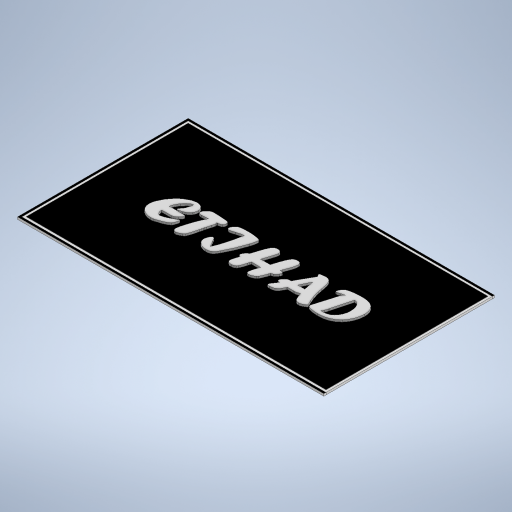
# Autodesk Inventor part: banner1
Saved by Autodesk Inventor 2024.1 (Build 281209000, 209)
## iProperties
Created: 2023-11-18
Part Number: banner1
Material: Generic
Document SubType Name: Modeling
Designer: ASUS
Density: 1 g/cm^3
Appearance: Default
Author: ASUS
Autodesk Inventor part; units mm, degrees
ref_plane "YZ Plane" through (0, 0, 0) normal (1, 0, 0) x (0, 1, 0)
ref_plane "XZ Plane" through (0, 0, 0) normal (0, 1, 0) x (-1, 0, 0)
ref_plane "XY Plane" through (0, 0, 0) normal (0, 0, 1) x (1, 0, 0)
sketch "Sketch1" plane through (0, 0, 0) normal (0, 1, 0) x (-1, 0, 0)
  line L0 (0, 0) -> (-71120, 0)
  line L1 (-71120, 0) -> (-71120, -19812)
  line L2 (-71120, -19812) -> (0, -19812)
  line L3 (0, -19812) -> (0, 0)
  line L4 (-254, -19558) -> (-70866, -19558)
  line L5 (-70866, -19558) -> (-70866, -254)
  line L6 (-70866, -254) -> (-254, -254)
  line L7 (-254, -254) -> (-254, -19558)
  line L8 (-35306, -19304) -> (-508, -19304)
  line L9 (-508, -19304) -> (-508, -508)
  line L10 (-508, -508) -> (-35306, -508)
  line L11 (-35306, -19304) -> (-35306, -508)
  line L12 (-6360.801, -11690.8525) -> (-20933.2375, -11690.8525) construction
  line L13 (-20933.2375, -11690.8525) -> (-20933.2375, -13635.6389) construction
  line L14 (-20933.2375, -13635.6389) -> (-6360.801, -13635.6389) construction
  line L15 (-6360.801, -13635.6389) -> (-6360.801, -11690.8525) construction
  line L16 (-41409.9422, -12220.6361) -> (-77079.4209, -12220.6361) construction
  line L17 (-77079.4209, -12220.6361) -> (-77079.4209, 7485.6525) construction
  line L18 (-77079.4209, 7485.6525) -> (-41409.9422, 7485.6525) construction
  line L19 (-41409.9422, 7485.6525) -> (-41409.9422, -12220.6361) construction
  line L20 (-9051.7121, -8799.8737) -> (-7938.0017, -8806.5427)
  line L21 (-7938.0017, -8806.5427) -> (-7938.0017, -8729.85)
  spline S0 degree 2 poles (-7938.0017, -8729.85) (-7938.0017, -8509.7755) (-8194.7553, -8146.3191) (-8351.475, -8146.3191) knots 0 0 0 1 2 2 2
  spline S1 degree 2 poles (-8351.475, -8146.3191) (-8508.1947, -8146.3191) (-9111.7324, -8379.7315) (-9495.1956, -8593.1371) knots 0 0 0 1 2 2 2
  line L22 (-9495.1956, -8593.1371) -> (-9601.8984, -8659.8263)
  spline S2 degree 2 poles (-9601.8984, -8659.8263) (-9711.9356, -8719.8466) (-9751.9492, -8749.8568) knots 0 0 0 1 1 1
  spline S3 degree 2 poles (-9751.9492, -8749.8568) (-9932.0102, -8863.2285) (-9978.6926, -8863.2285) knots 0 0 0 1 1 1
  spline S4 degree 2 poles (-9978.6926, -8863.2285) (-10032.044, -8863.2285) (-10032.044, -8763.1946) knots 0 0 0 1 1 1
  spline S5 degree 2 poles (-10032.044, -8763.1946) (-10032.044, -8653.1574) (-9952.0169, -8373.0625) (-9831.9763, -8112.9745) (-9768.6215, -8059.6231) knots 0 0 0 1 2 3 3 3
  spline S6 degree 2 poles (-9768.6215, -8059.6231) (-9595.2295, -7902.9034) (-8754.945, -7536.1125) (-8321.4648, -7432.7442) knots 0 0 0 1 2 2 2
  spline S7 degree 2 poles (-8321.4648, -7432.7442) (-8174.7485, -7402.734) (-8051.3734, -7402.734) knots 0 0 0 1 1 1
  spline S8 degree 2 poles (-8051.3734, -7402.734) (-7634.5656, -7402.734) (-6940.9974, -7739.5147) (-6560.8687, -8333.049) (-6560.8687, -8696.5054) knots 0 0 0 1 2 3 3 3
  spline S9 degree 2 poles (-6560.8687, -8696.5054) (-6560.8687, -8993.2725) (-6810.9534, -9713.5164) (-7261.1058, -10430.4258) (-7544.5351, -10720.524) knots 0 0 0 1 2 3 3 3
  spline S10 degree 2 poles (-7544.5351, -10720.524) (-7794.6198, -10977.2776) (-8404.8264, -11394.0854) (-8978.3539, -11620.8289) (-9221.7697, -11620.8289) knots 0 0 0 1 2 3 3 3
  spline S11 degree 2 poles (-9221.7697, -11620.8289) (-9598.5639, -11620.8289) (-10138.7468, -11190.6832) (-10138.7468, -10887.2471) knots 0 0 0 1 2 2 2
  spline S12 degree 2 poles (-10138.7468, -10887.2471) (-10138.7468, -10753.8687) (-10042.0474, -10437.0947) (-9958.6859, -10317.0541) knots 0 0 0 1 2 2 2
  spline S13 degree 2 poles (-9958.6859, -10317.0541) (-9871.9898, -10190.3445) (-9538.5436, -9946.9288) (-9328.4725, -9856.8983) knots 0 0 0 1 2 2 2
  spline S14 degree 2 poles (-9328.4725, -9856.8983) (-9075.0533, -9756.8644) (-8894.9924, -9756.8644) knots 0 0 0 1 1 1
  spline S15 degree 2 poles (-8894.9924, -9756.8644) (-8714.9314, -9756.8644) (-8714.9314, -9843.5604) knots 0 0 0 1 1 1
  spline S16 degree 2 poles (-8714.9314, -9843.5604) (-8714.9314, -9896.9118) (-8814.9653, -10006.9491) knots 0 0 0 1 1 1
  spline S17 degree 2 poles (-8814.9653, -10006.9491) (-8925.0025, -10103.6485) (-9025.0364, -10273.7061) knots 0 0 0 1 1 1
  spline S18 degree 2 poles (-9025.0364, -10273.7061) (-9121.7358, -10453.767) (-9268.4522, -10940.5985) (-9268.4522, -11077.3115) knots 0 0 0 1 2 2 2
  spline S19 degree 2 poles (-9268.4522, -11077.3115) (-9268.4522, -11190.6832) (-9201.7629, -11190.6832) knots 0 0 0 1 1 1
  spline S20 degree 2 poles (-9201.7629, -11190.6832) (-9095.0601, -11190.6832) (-8538.2049, -10720.524) (-8378.1507, -10493.7806) knots 0 0 0 1 2 2 2
  spline S21 degree 2 poles (-8378.1507, -10493.7806) (-8224.7654, -10280.375) (-8028.0322, -9836.8915) (-7994.6875, -9623.4859) knots 0 0 0 1 2 2 2
  line L23 (-7994.6875, -9623.4859) -> (-9625.2396, -9623.4859)
  spline S22 degree 2 poles (-9625.2396, -9623.4859) (-9895.3311, -9623.4859) (-9895.3311, -9486.773) knots 0 0 0 1 1 1
  spline S23 degree 2 poles (-9895.3311, -9486.773) (-9895.3311, -9356.7289) (-9595.2295, -9069.9652) knots 0 0 0 1 1 1
  spline S24 degree 2 poles (-9595.2295, -9069.9652) (-9298.4623, -8799.8737) (-9051.7121, -8799.8737) knots 0 0 0 1 1 1
  line L24 (-12172.7688, -9406.7459) -> (-12142.7587, -9273.3674)
  spline S25 degree 2 poles (-12142.7587, -9273.3674) (-12129.4208, -9206.6781) (-12102.7451, -9113.3132) (-12089.4073, -9043.2895) (-12079.4039, -9006.6104) knots 0 0 0 1 2 3 3 3
  spline S26 degree 2 poles (-12079.4039, -9006.6104) (-11859.3294, -8066.292) (-11725.9509, -7832.8796) knots 0 0 0 1 1 1
  spline S27 degree 2 poles (-11725.9509, -7832.8796) (-11665.9306, -7729.5113) (-11542.5555, -7646.1498) knots 0 0 0 1 1 1
  spline S28 degree 2 poles (-11542.5555, -7646.1498) (-11159.0923, -7396.0651) (-10939.0178, -7396.0651) knots 0 0 0 1 1 1
  spline S29 degree 2 poles (-10939.0178, -7396.0651) (-10785.6325, -7396.0651) (-10575.5614, -7619.4741) (-10575.5614, -7782.8627) knots 0 0 0 1 2 2 2
  spline S30 degree 2 poles (-10575.5614, -7782.8627) (-10575.5614, -8082.9643) (-10838.9839, -8886.5697) knots 0 0 0 1 1 1
  spline S31 degree 2 poles (-10838.9839, -8886.5697) (-10915.6765, -9143.3233) (-11049.055, -9520.1176) (-11232.4505, -9996.9457) (-11469.1973, -10533.7941) (-11515.8798, -10643.8314) knots 0 0 0 1 2 3 4 4 4
  spline S32 degree 2 poles (-11515.8798, -10643.8314) (-11115.7443, -10583.8111) (-10742.2845, -10583.8111) knots 0 0 0 1 1 1
  spline S33 degree 2 poles (-10742.2845, -10583.8111) (-10368.8247, -10583.8111) (-10368.8247, -10847.2336) knots 0 0 0 1 1 1
  spline S34 degree 2 poles (-10368.8247, -10847.2336) (-10368.8247, -11013.9567) (-10612.2405, -11270.7103) knots 0 0 0 1 1 1
  spline S35 degree 2 poles (-10612.2405, -11270.7103) (-10775.6291, -11440.7679) (-11055.724, -11570.8119) (-11255.7917, -11570.8119) knots 0 0 0 1 2 2 2
  spline S36 degree 2 poles (-11255.7917, -11570.8119) (-11382.5013, -11570.8119) (-11829.3192, -11554.1396) (-12222.7858, -11527.4639) knots 0 0 0 1 2 2 2
  line L25 (-12222.7858, -11527.4639) -> (-12309.4818, -11520.795)
  line L26 (-12309.4818, -11520.795) -> (-12389.5089, -11510.7916)
  spline S37 degree 2 poles (-12389.5089, -11510.7916) (-12726.2896, -11494.1193) (-12939.6952, -11444.1024) (-13016.3878, -11374.0787) knots 0 0 0 1 2 2 2
  spline S38 degree 2 poles (-13016.3878, -11374.0787) (-13076.4081, -11304.0549) (-13076.4081, -11214.0245) knots 0 0 0 1 1 1
  spline S39 degree 2 poles (-13076.4081, -11214.0245) (-13076.4081, -11117.3251) (-12999.7155, -10913.9228) (-12946.3641, -10863.9059) knots 0 0 0 1 2 2 2
  spline S40 degree 2 poles (-12946.3641, -10863.9059) (-12869.6715, -10780.5444) (-12519.5529, -10720.524) knots 0 0 0 1 1 1
  spline S41 degree 2 poles (-12519.5529, -10720.524) (-12489.5428, -10720.524) (-12456.1981, -10717.1896) knots 0 0 0 1 1 1
  line L27 (-12456.1981, -10717.1896) -> (-12392.8434, -10703.8517)
  spline S42 degree 2 poles (-12392.8434, -10703.8517) (-12466.2015, -10630.4935) (-12466.2015, -10540.4631) knots 0 0 0 1 1 1
  spline S43 degree 2 poles (-12466.2015, -10540.4631) (-12466.2015, -10457.1015) (-12382.84, -10173.6722) knots 0 0 0 1 1 1
  spline S44 degree 2 poles (-12382.84, -10173.6722) (-12352.8298, -10103.6485) (-12249.4615, -9713.5164) knots 0 0 0 1 1 1
  line L28 (-12249.4615, -9713.5164) -> (-12206.1135, -9530.121)
  line L29 (-12206.1135, -9530.121) -> (-12172.7688, -9406.7459)
  line L30 (-15307.1634, -11033.9635) -> (-15283.8222, -11033.9635)
  spline S45 degree 2 poles (-15283.8222, -11033.9635) (-15027.0686, -11033.9635) (-14430.1999, -10840.5647) knots 0 0 0 1 1 1
  spline S46 degree 2 poles (-14430.1999, -10840.5647) (-13990.0508, -10697.1828) (-13850.0034, -10697.1828) knots 0 0 0 1 1 1
  spline S47 degree 2 poles (-13850.0034, -10697.1828) (-13753.304, -10697.1828) (-13613.2566, -10820.5579) (-13613.2566, -10910.5884) knots 0 0 0 1 2 2 2
  spline S48 degree 2 poles (-13613.2566, -10910.5884) (-13613.2566, -11057.3047) (-13946.7028, -11487.4504) (-14113.4259, -11554.1396) knots 0 0 0 1 2 2 2
  spline S49 degree 2 poles (-14113.4259, -11554.1396) (-14360.1761, -11654.1735) (-15150.4437, -11654.1735) knots 0 0 0 1 1 1
  spline S50 degree 2 poles (-15150.4437, -11654.1735) (-15463.8832, -11654.1735) (-16097.431, -11594.1532) (-16534.2456, -11487.4504) (-16594.2659, -11427.43) knots 0 0 0 1 2 3 3 3
  spline S51 degree 2 poles (-16594.2659, -11427.43) (-16624.2761, -11397.4199) (-16624.2761, -11297.386) knots 0 0 0 1 1 1
  spline S52 degree 2 poles (-16624.2761, -11297.386) (-16624.2761, -11204.0211) (-16524.2422, -10723.8585) (-16454.2185, -10507.1184) knots 0 0 0 1 2 2 2
  spline S53 degree 2 poles (-16454.2185, -10507.1184) (-16024.0728, -9163.3301) (-15437.2075, -8089.6332) knots 0 0 0 1 1 1
  spline S54 degree 2 poles (-15437.2075, -8089.6332) (-15290.4911, -7819.5418) (-15020.3997, -7526.1091) (-14693.6224, -7402.734) (-14466.8789, -7402.734) knots 0 0 0 1 2 3 3 3
  spline S55 degree 2 poles (-14466.8789, -7402.734) (-14143.4361, -7402.734) (-13589.9153, -7649.4842) (-13269.807, -8072.9609) (-13269.807, -8326.3801) knots 0 0 0 1 2 3 3 3
  spline S56 degree 2 poles (-13269.807, -8326.3801) (-13269.807, -8503.1066) (-13419.8578, -8909.911) (-13513.2227, -9019.9482) knots 0 0 0 1 2 2 2
  spline S57 degree 2 poles (-13513.2227, -9019.9482) (-13559.9052, -9076.6341) (-13619.9255, -9076.6341) knots 0 0 0 1 1 1
  spline S58 degree 2 poles (-13619.9255, -9076.6341) (-13719.9594, -9076.6341) (-13896.6859, -8886.5697) (-14003.3887, -8659.8263) knots 0 0 0 1 2 2 2
  spline S59 degree 2 poles (-14003.3887, -8659.8263) (-14150.105, -8313.0422) (-14343.5038, -8082.9643) knots 0 0 0 1 1 1
  spline S60 degree 2 poles (-14343.5038, -8082.9643) (-14363.5106, -8056.2886) (-14436.8688, -7976.2615) knots 0 0 0 1 1 1
  spline S61 degree 2 poles (-14436.8688, -7976.2615) (-14580.2507, -8296.3699) (-14736.9704, -8706.5088) (-14837.0043, -9053.2929) knots 0 0 0 1 2 2 2
  spline S62 degree 2 poles (-14837.0043, -9053.2929) (-14907.028, -9270.0329) (-15073.7511, -9900.2463) knots 0 0 0 1 1 1
  spline S63 degree 2 poles (-15073.7511, -9900.2463) (-15207.1296, -10427.0913) (-15307.1634, -11033.9635) knots 0 0 0 1 1 1
  line L31 (-18364.8654, -8793.2048) -> (-18301.5106, -8589.8026)
  spline S64 degree 2 poles (-18301.5106, -8589.8026) (-18288.1728, -8523.1134) (-18254.8282, -8409.7416) knots 0 0 0 1 1 1
  spline S65 degree 2 poles (-18254.8282, -8409.7416) (-18088.105, -7836.2141) (-17981.4022, -7656.1531) knots 0 0 0 1 1 1
  spline S66 degree 2 poles (-17981.4022, -7656.1531) (-17958.061, -7619.4741) (-17901.3751, -7549.4503) knots 0 0 0 1 1 1
  spline S67 degree 2 poles (-17901.3751, -7549.4503) (-17704.6419, -7369.3894) (-17421.2126, -7369.3894) knots 0 0 0 1 1 1
  spline S68 degree 2 poles (-17421.2126, -7369.3894) (-17194.4691, -7369.3894) (-16921.0432, -7566.1227) (-16921.0432, -7722.8424) knots 0 0 0 1 2 2 2
  spline S69 degree 2 poles (-16921.0432, -7722.8424) (-16921.0432, -7836.2141) (-17081.0974, -8416.4106) (-17177.7968, -8679.8331) knots 0 0 0 1 2 2 2
  spline S70 degree 2 poles (-17177.7968, -8679.8331) (-16937.7155, -8726.5156) (-16937.7155, -8883.2353) knots 0 0 0 1 1 1
  spline S71 degree 2 poles (-16937.7155, -8883.2353) (-16937.7155, -8996.607) (-17087.7663, -9280.0363) (-17314.5098, -9506.7797) (-17421.2126, -9540.1244) knots 0 0 0 1 2 3 3 3
  spline S72 degree 2 poles (-17421.2126, -9540.1244) (-17467.895, -9670.1684) (-17597.9391, -10090.3107) knots 0 0 0 1 1 1
  spline S73 degree 2 poles (-17597.9391, -10090.3107) (-17884.7028, -11003.9533) (-18064.7638, -11314.0583) knots 0 0 0 1 1 1
  spline S74 degree 2 poles (-18064.7638, -11314.0583) (-18138.122, -11417.4267) (-18191.4734, -11474.1125) knots 0 0 0 1 1 1
  spline S75 degree 2 poles (-18191.4734, -11474.1125) (-18348.1931, -11624.1633) (-18594.9433, -11624.1633) knots 0 0 0 1 1 1
  spline S76 degree 2 poles (-18594.9433, -11624.1633) (-18748.3286, -11624.1633) (-18981.7409, -11517.4605) (-19105.116, -11330.7306) (-19105.116, -11207.3555) knots 0 0 0 1 2 3 3 3
  spline S77 degree 2 poles (-19105.116, -11207.3555) (-19105.116, -11033.9635) (-18671.6359, -9746.861) knots 0 0 0 1 1 1
  spline S78 degree 2 poles (-18671.6359, -9746.861) (-18664.967, -9726.8543) (-18638.2913, -9643.4927) (-18624.9535, -9610.1481) knots 0 0 0 1 2 2 2
  line L32 (-18624.9535, -9610.1481) -> (-18614.9501, -9586.8068)
  line L33 (-18614.9501, -9586.8068) -> (-19735.3294, -9610.1481)
  line L34 (-19735.3294, -9610.1481) -> (-19788.6808, -9803.5469)
  spline S79 degree 2 poles (-19788.6808, -9803.5469) (-19885.3802, -10113.6519) (-20092.1169, -10720.524) (-20242.1677, -11087.3149) (-20395.553, -11367.4097) (-20462.2422, -11437.4334) knots 0 0 0 1 2 3 4 4 4
  spline S80 degree 2 poles (-20462.2422, -11437.4334) (-20622.2964, -11610.8255) (-20902.3912, -11610.8255) knots 0 0 0 1 1 1
  spline S81 degree 2 poles (-20902.3912, -11610.8255) (-21375.8849, -11610.8255) (-21375.8849, -11200.6866) knots 0 0 0 1 1 1
  spline S82 degree 2 poles (-21375.8849, -11200.6866) (-21375.8849, -10813.889) (-20962.4116, -9790.209) knots 0 0 0 1 1 1
  spline S83 degree 2 poles (-20962.4116, -9790.209) (-20902.3912, -9636.8238) (-20892.3879, -9603.4791) knots 0 0 0 1 1 1
  spline S84 degree 2 poles (-20892.3879, -9603.4791) (-20902.3912, -9606.8136) (-20922.398, -9610.1481) (-20932.4014, -9610.1481) knots 0 0 0 1 2 2 2
  spline S85 degree 2 poles (-20932.4014, -9610.1481) (-21099.1245, -9610.1481) (-21289.1889, -9490.1074) (-21289.1889, -9390.0736) knots 0 0 0 1 2 2 2
  spline S86 degree 2 poles (-21289.1889, -9390.0736) (-21289.1889, -9323.3843) (-21205.8273, -9196.6747) knots 0 0 0 1 1 1
  spline S87 degree 2 poles (-21205.8273, -9196.6747) (-21125.8002, -9073.2996) (-20939.0703, -8879.9008) (-20872.3811, -8839.8873) knots 0 0 0 1 2 2 2
  spline S88 degree 2 poles (-20872.3811, -8839.8873) (-20809.0263, -8806.5427) (-20625.6309, -8769.8636) knots 0 0 0 1 1 1
  line L35 (-20625.6309, -8769.8636) -> (-20612.293, -8719.8466)
  spline S89 degree 2 poles (-20612.293, -8719.8466) (-20592.2862, -8676.4986) (-20548.9382, -8553.1235) knots 0 0 0 1 1 1
  spline S90 degree 2 poles (-20548.9382, -8553.1235) (-20485.5835, -8376.397) (-20352.205, -8019.6095) (-20262.1745, -7822.8763) (-20218.8265, -7756.187) knots 0 0 0 1 2 3 3 3
  spline S91 degree 2 poles (-20218.8265, -7756.187) (-20168.8095, -7682.8288) (-20102.1203, -7632.8119) knots 0 0 0 1 1 1
  spline S92 degree 2 poles (-20102.1203, -7632.8119) (-19955.4039, -7519.4402) (-19575.2752, -7376.0583) (-19451.9001, -7376.0583) knots 0 0 0 1 2 2 2
  spline S93 degree 2 poles (-19451.9001, -7376.0583) (-19305.1838, -7376.0583) (-19141.7951, -7516.1057) (-19141.7951, -7642.8153) knots 0 0 0 1 2 2 2
  spline S94 degree 2 poles (-19141.7951, -7642.8153) (-19141.7951, -7862.8898) (-19371.873, -8553.1235) knots 0 0 0 1 1 1
  spline S95 degree 2 poles (-19371.873, -8553.1235) (-19425.2244, -8706.5088) (-19445.2312, -8776.5325) knots 0 0 0 1 1 1
  line L36 (-19445.2312, -8776.5325) -> (-18364.8654, -8793.2048)
  line L37 (-23676.6639, -11133.9974) -> (-23489.934, -11467.4436)
  spline S96 degree 2 poles (-23489.934, -11467.4436) (-23559.9577, -11524.1295) (-23619.9781, -11544.1362) knots 0 0 0 1 1 1
  spline S97 degree 2 poles (-23619.9781, -11544.1362) (-23856.7249, -11624.1633) (-24186.8366, -11624.1633) knots 0 0 0 1 1 1
  spline S98 degree 2 poles (-24186.8366, -11624.1633) (-24523.6173, -11624.1633) (-24707.0128, -11430.7645) knots 0 0 0 1 1 1
  spline S99 degree 2 poles (-24707.0128, -11430.7645) (-24863.7325, -11264.0414) (-25063.8002, -10660.5037) (-25150.4963, -10103.6485) knots 0 0 0 1 2 2 2
  spline S100 degree 2 poles (-25150.4963, -10103.6485) (-25197.1787, -9820.2192) (-25230.5234, -9676.8373) knots 0 0 0 1 1 1
  spline S101 degree 2 poles (-25230.5234, -9676.8373) (-25337.2262, -9276.7018) (-25407.2499, -9056.6273) (-25500.6148, -8813.2116) knots 0 0 0 1 2 2 2
  spline S102 degree 2 poles (-25500.6148, -8813.2116) (-25530.625, -8743.1879) (-25630.6588, -8489.7687) (-25677.3413, -8379.7315) knots 0 0 0 1 2 2 2
  spline S103 degree 2 poles (-25677.3413, -8379.7315) (-25777.3752, -8142.9846) (-25980.7774, -7752.8526) knots 0 0 0 1 1 1
  spline S104 degree 2 poles (-25980.7774, -7752.8526) (-25724.0238, -7572.7916) (-25370.5708, -7412.7374) (-25223.8544, -7412.7374) knots 0 0 0 1 2 2 2
  spline S105 degree 2 poles (-25223.8544, -7412.7374) (-25043.7935, -7412.7374) (-24803.7122, -7552.7848) (-24707.0128, -7706.1701) knots 0 0 0 1 2 2 2
  spline S106 degree 2 poles (-24707.0128, -7706.1701) (-24590.3066, -7912.9067) (-24473.6004, -8269.6942) knots 0 0 0 1 1 1
  spline S107 degree 2 poles (-24473.6004, -8269.6942) (-24463.597, -8303.0388) (-24430.2524, -8406.4072) (-24406.9112, -8469.762) knots 0 0 0 1 2 2 2
  spline S108 degree 2 poles (-24406.9112, -8469.762) (-24050.1237, -8319.7111) (-23853.3904, -8319.7111) knots 0 0 0 1 1 1
  spline S109 degree 2 poles (-23853.3904, -8319.7111) (-23740.0187, -8319.7111) (-23656.6571, -8326.3801) knots 0 0 0 1 1 1
  spline S110 degree 2 poles (-23656.6571, -8326.3801) (-23586.6334, -8329.7145) (-23003.1025, -8343.0524) knots 0 0 0 1 1 1
  line L38 (-23003.1025, -8343.0524) -> (-22976.4268, -8283.0321)
  spline S111 degree 2 poles (-22976.4268, -8283.0321) (-22806.3692, -7926.2446) (-22516.271, -7552.7848) (-22132.8078, -7399.3995) (-21846.0441, -7399.3995) knots 0 0 0 1 2 3 3 3
  spline S112 degree 2 poles (-21846.0441, -7399.3995) (-21682.6554, -7399.3995) (-21542.608, -7472.7577) (-21542.608, -7556.1193) knots 0 0 0 1 2 2 2
  spline S113 degree 2 poles (-21542.608, -7556.1193) (-21542.608, -7656.1531) (-21879.3887, -8109.64) knots 0 0 0 1 1 1
  spline S114 degree 2 poles (-21879.3887, -8109.64) (-21996.0949, -8269.6942) (-22056.1152, -8359.7247) knots 0 0 0 1 1 1
  spline S115 degree 2 poles (-22056.1152, -8359.7247) (-21736.0068, -8419.745) (-21736.0068, -8586.4681) knots 0 0 0 1 1 1
  spline S116 degree 2 poles (-21736.0068, -8586.4681) (-21736.0068, -8719.8466) (-21992.7604, -8986.6036) knots 0 0 0 1 1 1
  spline S117 degree 2 poles (-21992.7604, -8986.6036) (-22112.8011, -9113.3132) (-22322.8722, -9183.3369) (-22586.2947, -9186.6714) knots 0 0 0 1 2 2 2
  spline S118 degree 2 poles (-22586.2947, -9186.6714) (-22829.7105, -9633.4893) (-22963.089, -9880.2395) (-23176.4946, -10257.0338) (-23446.586, -10733.8619) (-23676.6639, -11133.9974) knots 0 0 0 1 2 3 4 4 4
  line L39 (-23940.0864, -10327.0575) -> (-23383.2312, -9146.6578)
  line L40 (-23383.2312, -9146.6578) -> (-24206.8434, -9146.6578)
  line L41 (-24206.8434, -9146.6578) -> (-23950.0898, -10327.0575)
  line L42 (-23950.0898, -10327.0575) -> (-23940.0864, -10327.0575)
  line L43 (-26137.4971, -7919.5757) -> (-26864.4099, -10367.071)
  spline S119 degree 2 poles (-26864.4099, -10367.071) (-26941.1025, -10650.5003) (-27024.4641, -10767.2065) knots 0 0 0 1 1 1
  spline S120 degree 2 poles (-27024.4641, -10767.2065) (-27077.8155, -10833.8958) (-27161.1771, -10880.5782) knots 0 0 0 1 1 1
  line L44 (-27161.1771, -10880.5782) -> (-27161.1771, -10890.5816)
  line L45 (-27161.1771, -10890.5816) -> (-27117.829, -10890.5816)
  spline S121 degree 2 poles (-27117.829, -10890.5816) (-27031.133, -10890.5816) (-26751.0382, -10790.5477) knots 0 0 0 1 1 1
  spline S122 degree 2 poles (-26751.0382, -10790.5477) (-26444.2677, -10683.8449) (-26327.5615, -10683.8449) knots 0 0 0 1 1 1
  spline S123 degree 2 poles (-26327.5615, -10683.8449) (-26267.5411, -10683.8449) (-26220.8587, -10727.193) (-26220.8587, -10777.2099) knots 0 0 0 1 2 2 2
  spline S124 degree 2 poles (-26220.8587, -10777.2099) (-26220.8587, -10900.585) (-26357.5716, -11190.6832) (-26577.6461, -11420.7611) (-26694.3523, -11470.7781) knots 0 0 0 1 2 3 3 3
  spline S125 degree 2 poles (-26694.3523, -11470.7781) (-26957.7749, -11574.1464) (-27864.7486, -11690.8526) (-28398.2626, -11690.8526) knots 0 0 0 1 2 2 2
  spline S126 degree 2 poles (-28398.2626, -11690.8526) (-28971.7901, -11690.8526) (-29775.3955, -11330.7306) (-30192.2033, -10623.8246) (-30192.2033, -10123.6553) knots 0 0 0 1 2 3 3 3
  spline S127 degree 2 poles (-30192.2033, -10123.6553) (-30192.2033, -9620.1515) (-29792.0678, -8599.806) (-29465.2905, -8253.0219) knots 0 0 0 1 2 2 2
  spline S128 degree 2 poles (-29465.2905, -8253.0219) (-28695.0297, -7436.0786) (-27404.5928, -7436.0786) knots 0 0 0 1 1 1
  spline S129 degree 2 poles (-27404.5928, -7436.0786) (-26991.1195, -7436.0786) (-26304.2202, -7569.4571) (-26194.183, -7669.491) knots 0 0 0 1 2 2 2
  spline S130 degree 2 poles (-26194.183, -7669.491) (-26124.1593, -7722.8424) (-26124.1593, -7829.5452) knots 0 0 0 1 1 1
  spline S131 degree 2 poles (-26124.1593, -7829.5452) (-26124.1593, -7856.2209) (-26137.4971, -7919.5757) knots 0 0 0 1 1 1
  line L46 (-28201.5293, -10953.9364) -> (-27584.6538, -8636.4851)
  spline S132 degree 2 poles (-27584.6538, -8636.4851) (-27577.9848, -8613.1438) (-27561.3125, -8523.1134) knots 0 0 0 1 1 1
  spline S133 degree 2 poles (-27561.3125, -8523.1134) (-27504.6267, -8283.0321) (-27434.603, -8149.6536) knots 0 0 0 1 1 1
  spline S134 degree 2 poles (-27434.603, -8149.6536) (-27387.9205, -8049.6197) (-27281.2177, -7919.5757) knots 0 0 0 1 1 1
  spline S135 degree 2 poles (-27281.2177, -7919.5757) (-27367.9137, -7912.9067) (-27477.951, -7912.9067) knots 0 0 0 1 1 1
  spline S136 degree 2 poles (-27477.951, -7912.9067) (-27744.708, -7912.9067) (-28098.161, -7982.9305) (-28401.597, -8152.988) (-28534.9755, -8289.701) knots 0 0 0 1 2 3 3 3
  spline S137 degree 2 poles (-28534.9755, -8289.701) (-28788.3947, -8546.4546) (-29058.4861, -9230.0194) (-29058.4861, -9630.1548) knots 0 0 0 1 2 2 2
  spline S138 degree 2 poles (-29058.4861, -9630.1548) (-29058.4861, -9996.9457) (-28841.7461, -10593.8145) (-28451.614, -10937.2641) (-28201.5293, -10953.9364) knots 0 0 0 1 2 3 3 3
  spline S139 degree 2 poles (-42991.5474, -7910.8463) (-42539.6602, -7910.8463) (-41905.6692, -8099.6946) (-41625.769, -8234.5863) knots 0 0 0 1 2 2 2
  line L47 (-41625.769, -8234.5863) -> (-41625.769, -8929.2786)
  line L48 (-41625.769, -8929.2786) -> (-41666.2365, -8929.2786)
  spline S140 degree 2 poles (-41666.2365, -8929.2786) (-41939.3922, -8672.9844) (-42630.7121, -8389.7118) (-42951.0799, -8389.7118) knots 0 0 0 1 2 2 2
  spline S141 degree 2 poles (-42951.0799, -8389.7118) (-43409.7117, -8389.7118) (-43878.4604, -8770.7809) (-43878.4604, -9084.4041) knots 0 0 0 1 2 2 2
  spline S142 degree 2 poles (-43878.4604, -9084.4041) (-43878.4604, -9333.9537) (-43632.283, -9644.2046) (-43365.8719, -9721.7673) knots 0 0 0 1 2 2 2
  spline S143 degree 2 poles (-43365.8719, -9721.7673) (-43173.6512, -9775.724) (-42853.2834, -9849.9145) (-42613.8507, -9910.6157) knots 0 0 0 1 2 2 2
  spline S144 degree 2 poles (-42613.8507, -9910.6157) (-42398.024, -9967.9447) (-42057.4224, -10139.9316) (-41925.903, -10278.1956) knots 0 0 0 1 2 2 2
  spline S145 degree 2 poles (-41925.903, -10278.1956) (-41797.7559, -10416.4596) (-41656.1196, -10787.4118) (-41656.1196, -11030.2169) knots 0 0 0 1 2 2 2
  spline S146 degree 2 poles (-41656.1196, -11030.2169) (-41656.1196, -11536.0607) (-42445.236, -12220.6361) (-43055.621, -12220.6361) knots 0 0 0 1 2 2 2
  spline S147 degree 2 poles (-43055.621, -12220.6361) (-43406.3394, -12220.6361) (-44026.8413, -12082.3721) (-44293.2524, -11950.8527) knots 0 0 0 1 2 2 2
  line L49 (-44293.2524, -11950.8527) -> (-44293.2524, -11289.8834)
  line L50 (-44293.2524, -11289.8834) -> (-44252.7849, -11289.8834)
  spline S148 degree 2 poles (-44252.7849, -11289.8834) (-44053.8196, -11471.9872) (-43433.3178, -11741.7706) (-43092.7162, -11741.7706) knots 0 0 0 1 2 2 2
  spline S149 degree 2 poles (-43092.7162, -11741.7706) (-42708.2749, -11741.7706) (-42232.7816, -11380.9353) (-42232.7816, -11087.5458) knots 0 0 0 1 2 2 2
  spline S150 degree 2 poles (-42232.7816, -11087.5458) (-42232.7816, -10824.507) (-42512.6819, -10510.8838) (-42775.7207, -10440.0657) knots 0 0 0 1 2 2 2
  spline S151 degree 2 poles (-42775.7207, -10440.0657) (-42951.0799, -10392.8536) (-43460.2961, -10271.451) (-43628.9107, -10220.8666) knots 0 0 0 1 2 2 2
  spline S152 degree 2 poles (-43628.9107, -10220.8666) (-44057.1919, -10089.3472) (-44455.1224, -9559.8973) (-44455.1224, -9172.0837) knots 0 0 0 1 2 2 2
  spline S153 degree 2 poles (-44455.1224, -9172.0837) (-44455.1224, -8925.9063) (-44256.1571, -8453.7854) (-44077.4256, -8288.543) knots 0 0 0 1 2 2 2
  spline S154 degree 2 poles (-44077.4256, -8288.543) (-43878.4604, -8106.4392) (-43372.6165, -7910.8463) (-42991.5474, -7910.8463) knots 0 0 0 1 2 2 2
  line L51 (-45989.5155, -7985.0367) -> (-45989.5155, -11654.091)
  line L52 (-45989.5155, -11654.091) -> (-44593.3864, -11654.091)
  line L53 (-44593.3864, -11654.091) -> (-44593.3864, -12146.4457)
  line L54 (-44593.3864, -12146.4457) -> (-47938.7006, -12146.4457)
  line L55 (-47938.7006, -12146.4457) -> (-47938.7006, -11654.091)
  line L56 (-47938.7006, -11654.091) -> (-46542.5715, -11654.091)
  line L57 (-46542.5715, -11654.091) -> (-46542.5715, -7985.0367)
  line L58 (-46542.5715, -7985.0367) -> (-45989.5155, -7985.0367)
  line L59 (-47911.7223, -7985.0367) -> (-49314.596, -12146.4457)
  line L60 (-49314.596, -12146.4457) -> (-49995.799, -12146.4457)
  line L61 (-49995.799, -12146.4457) -> (-51398.6727, -7985.0367)
  line L62 (-51398.6727, -7985.0367) -> (-50815.2661, -7985.0367)
  line L63 (-50815.2661, -7985.0367) -> (-50437.5694, -9148.4776)
  line L64 (-50437.5694, -9148.4776) -> (-48849.2196, -9148.4776)
  line L65 (-48849.2196, -9148.4776) -> (-48471.5228, -7985.0367)
  line L66 (-48471.5228, -7985.0367) -> (-47911.7223, -7985.0367)
  line L67 (-50285.8162, -9620.5986) -> (-49641.7083, -11579.9005)
  line L68 (-49641.7083, -11579.9005) -> (-49000.9727, -9620.5986)
  line L69 (-49000.9727, -9620.5986) -> (-50285.8162, -9620.5986)
  spline S155 degree 2 poles (-55074.4716, -10062.3689) (-55074.4716, -9492.4515) (-54612.4675, -8575.1879) (-54224.6539, -8318.8936) knots 0 0 0 1 2 2 2
  spline S156 degree 2 poles (-54224.6539, -8318.8936) (-53907.6584, -8119.9284) (-53256.8059, -7985.0367) (-52750.9621, -7985.0367) knots 0 0 0 1 2 2 2
  line L70 (-52750.9621, -7985.0367) -> (-51793.231, -7985.0367)
  line L71 (-51793.231, -7985.0367) -> (-51793.231, -12146.4457)
  line L72 (-51793.231, -12146.4457) -> (-52740.8452, -12146.4457)
  spline S157 degree 2 poles (-52740.8452, -12146.4457) (-53327.6241, -12146.4457) (-53995.338, -11971.0865) (-54231.3985, -11815.961) knots 0 0 0 1 2 2 2
  spline S158 degree 2 poles (-54231.3985, -11815.961) (-54632.7013, -11549.5499) (-55074.4716, -10669.3816) (-55074.4716, -10062.3689) knots 0 0 0 1 2 2 2
  spline S159 degree 2 poles (-54497.8096, -10069.1135) (-54497.8096, -10547.979) (-54180.8141, -11225.8098) (-53867.1909, -11418.0305) knots 0 0 0 1 2 2 2
  spline S160 degree 2 poles (-53867.1909, -11418.0305) (-53644.6196, -11549.5499) (-53142.148, -11667.5801) (-52767.8235, -11667.5801) knots 0 0 0 1 2 2 2
  line L73 (-52767.8235, -11667.5801) -> (-52346.287, -11667.5801)
  line L74 (-52346.287, -11667.5801) -> (-52346.287, -8463.9022)
  line L75 (-52346.287, -8463.9022) -> (-52767.8235, -8463.9022)
  spline S161 degree 2 poles (-52767.8235, -8463.9022) (-53135.4034, -8463.9022) (-53691.8317, -8581.9325) (-53917.7753, -8740.4302) knots 0 0 0 1 2 2 2
  spline S162 degree 2 poles (-53917.7753, -8740.4302) (-54207.7924, -8936.0232) (-54497.8096, -9583.5034) (-54497.8096, -10069.1135) knots 0 0 0 1 2 2 2
  line L76 (-57124.8255, -7985.0367) -> (-55512.8696, -7985.0367)
  line L77 (-55512.8696, -7985.0367) -> (-55512.8696, -8409.9455)
  line L78 (-55512.8696, -8409.9455) -> (-56042.3196, -8409.9455)
  line L79 (-56042.3196, -8409.9455) -> (-56042.3196, -11721.5368)
  line L80 (-56042.3196, -11721.5368) -> (-55512.8696, -11721.5368)
  line L81 (-55512.8696, -11721.5368) -> (-55512.8696, -12146.4457)
  line L82 (-55512.8696, -12146.4457) -> (-57124.8255, -12146.4457)
  line L83 (-57124.8255, -12146.4457) -> (-57124.8255, -11721.5368)
  line L84 (-57124.8255, -11721.5368) -> (-56595.3756, -11721.5368)
  line L85 (-56595.3756, -11721.5368) -> (-56595.3756, -8409.9455)
  line L86 (-56595.3756, -8409.9455) -> (-57124.8255, -8409.9455)
  line L87 (-57124.8255, -8409.9455) -> (-57124.8255, -7985.0367)
  spline S163 degree 2 poles (-59262.859, -7897.3571) (-58895.2791, -7897.3571) (-58348.9677, -8089.5778) (-58156.747, -8281.7984) knots 0 0 0 1 2 2 2
  spline S164 degree 2 poles (-58156.747, -8281.7984) (-57937.548, -8497.6252) (-57758.8165, -9104.6378) (-57758.8165, -9549.7804) knots 0 0 0 1 2 2 2
  line L88 (-57758.8165, -9549.7804) -> (-57758.8165, -12146.4457)
  line L89 (-57758.8165, -12146.4457) -> (-58311.8725, -12146.4457)
  line L90 (-58311.8725, -12146.4457) -> (-58311.8725, -9549.7804)
  spline S165 degree 2 poles (-58311.8725, -9549.7804) (-58311.8725, -9259.7633) (-58386.0629, -8868.5773) (-58490.604, -8710.0796) knots 0 0 0 1 2 2 2
  spline S166 degree 2 poles (-58490.604, -8710.0796) (-58601.8896, -8541.465) (-58986.331, -8369.478) (-59262.859, -8369.478) knots 0 0 0 1 2 2 2
  spline S167 degree 2 poles (-59262.859, -8369.478) (-59522.5255, -8369.478) (-59927.2006, -8541.465) (-60038.4862, -8710.0796) knots 0 0 0 1 2 2 2
  spline S168 degree 2 poles (-60038.4862, -8710.0796) (-60143.0273, -8868.5773) (-60217.2177, -9256.391) (-60217.2177, -9536.2913) knots 0 0 0 1 2 2 2
  line L91 (-60217.2177, -9536.2913) -> (-60217.2177, -12146.4457)
  line L92 (-60217.2177, -12146.4457) -> (-60770.2737, -12146.4457)
  line L93 (-60770.2737, -12146.4457) -> (-60770.2737, -9549.7804)
  spline S169 degree 2 poles (-60770.2737, -9549.7804) (-60770.2737, -9114.7547) (-60594.9145, -8494.2529) (-60372.3432, -8281.7984) knots 0 0 0 1 2 2 2
  spline S170 degree 2 poles (-60372.3432, -8281.7984) (-60173.3779, -8086.2055) (-59647.3003, -7897.3571) (-59262.859, -7897.3571) knots 0 0 0 1 2 2 2
  line L94 (-65130.648, -7985.0367) -> (-64577.592, -7985.0367)
  line L95 (-64577.592, -7985.0367) -> (-64577.592, -11569.7837)
  line L96 (-64577.592, -11569.7837) -> (-63491.7138, -9131.6162)
  line L97 (-63491.7138, -9131.6162) -> (-63154.4845, -9131.6162)
  line L98 (-63154.4845, -9131.6162) -> (-62078.7232, -11569.7837)
  line L99 (-62078.7232, -11569.7837) -> (-62078.7232, -7985.0367)
  line L100 (-62078.7232, -7985.0367) -> (-61562.7625, -7985.0367)
  line L101 (-61562.7625, -7985.0367) -> (-61562.7625, -12146.4457)
  line L102 (-61562.7625, -12146.4457) -> (-62318.156, -12146.4457)
  line L103 (-62318.156, -12146.4457) -> (-63356.8221, -9829.6807)
  line L104 (-63356.8221, -9829.6807) -> (-64361.7653, -12146.4457)
  line L105 (-64361.7653, -12146.4457) -> (-65130.648, -12146.4457)
  line L106 (-65130.648, -12146.4457) -> (-65130.648, -7985.0367)
  dimension "d3" = 19812
  constraints: 24 end point, 5 parallel, 2 perpendicular, 1 horizontal, 7 other
  measures "d3" distance of L0.end L1.end
extrude "Extrusion1" add sketch "Sketch1" along normal blind 508 contours L20 L21 S0 S1 L22 S2 S3 S4 S5 S6 S7 S8 S9 S10 S11 S12 S13 S14 S15 S16 S17 S18 S19 S20 S21 L23 S22 S23 S24 | L24 S25 S26 S27 S28 S29 S30 S31 S32 S33 S34 S35 S36 L25 L26 S37 S38 S39 S40 S41 L27 S42 S43 S44 L28 L29 | L30 S45 S46 S47 S48 S49 S50 S51 S52 S53 S54 S55 S56 S57 S58 S59 S60 S61 S62 S63 | L31 S64 S65 S66 S67 S68 S69 S70 S71 S72 S73 S74 S75 S76 S77 S78 L32 L33 L34 S79 S80 S81 S82 S83 S84 S85 S86 S87 S88 L35 S89 S90 S91 S92 S93 S94 S95 L36 | L37 S96 S97 S98 S99 S100 S101 S102 S103 S104 S105 S106 S107 S108 S109 S110 L38 S111 S112 S113 S114 S115 S116 S117 S118 | L43 S119 S120 L44 L45 S121 S122 S123 S124 S125 S126 S127 S128 S129 S130 S131
extrude "Extrusion2" add sketch "Sketch1" along normal blind 508 contours S139 L47 L48 S140 S141 S142 S143 S144 S145 S146 S147 L49 L50 S148 S149 S150 S151 S152 S153 S154 | L51 L52 L53 L54 L55 L56 L57 L58 | L59 L60 L61 L62 L63 L64 L65 L66 | S155 S156 L70 L71 L72 S157 S158 | L76 L77 L78 L79 L80 L81 L82 L83 L84 L85 L86 L87 | S163 S164 L88 L89 L90 S165 S166 S167 S168 L91 L92 L93 S169 S170 | L94 L95 L96 L97 L98 L99 L100 L101 L102 L103 L104 L105 L106
extrude "Extrusion3" cut sketch "Sketch1" along normal blind 254 contours L11 L10 L9 L8 | L20 L21 S0 S1 L22 S2 S3 S4 S5 S6 S7 S8 S9 S10 S11 S12 S13 S14 S15 S16 S17 S18 S19 S20 S21 L23 S22 S23 S24 | L24 S25 S26 S27 S28 S29 S30 S31 S32 S33 S34 S35 S36 L25 L26 S37 S38 S39 S40 S41 L27 S42 S43 S44 L28 L29 | L30 S45 S46 S47 S48 S49 S50 S51 S52 S53 S54 S55 S56 S57 S58 S59 S60 S61 S62 S63 | L31 S64 S65 S66 S67 S68 S69 S70 S71 S72 S73 S74 S75 S76 S77 S78 L32 L33 L34 S79 S80 S81 S82 S83 S84 S85 S86 S87 S88 L35 S89 S90 S91 S92 S93 S94 S95 L36 | L37 S96 S97 S98 S99 S100 S101 S102 S103 S104 S105 S106 S107 S108 S109 S110 L38 S111 S112 S113 S114 S115 S116 S117 S118 | L42 L41 L40 L39 | L43 S119 S120 L44 L45 S121 S122 S123 S124 S125 S126 S127 S128 S129 S130 S131 | S138 S137 S136 S135 S134 S133 S132 L46
extrude "Extrusion4" cut sketch "Sketch1" along normal blind 254 contours L4 L5 L6 L7 | S139 L47 L48 S140 S141 S142 S143 S144 S145 S146 S147 L49 L50 S148 S149 S150 S151 S152 S153 S154 | L51 L52 L53 L54 L55 L56 L57 L58 | L59 L60 L61 L62 L63 L64 L65 L66 | L69 L68 L67 | S155 S156 L70 L71 L72 S157 S158 | S162 S161 L75 L74 L73 S160 S159 | L76 L77 L78 L79 L80 L81 L82 L83 L84 L85 L86 L87 | S163 S164 L88 L89 L90 S165 S166 S167 S168 L91 L92 L93 S169 S170 | L94 L95 L96 L97 L98 L99 L100 L101 L102 L103 L104 L105 L106
extrude "Extrusion5" add sketch "Sketch1" along normal blind 254 contours L4 L5 L6 L7 | S139 L47 L48 S140 S141 S142 S143 S144 S145 S146 S147 L49 L50 S148 S149 S150 S151 S152 S153 S154 | L51 L52 L53 L54 L55 L56 L57 L58 | L59 L60 L61 L62 L63 L64 L65 L66 | L69 L68 L67 | S155 S156 L70 L71 L72 S157 S158 | S162 S161 L75 L74 L73 S160 S159 | L76 L77 L78 L79 L80 L81 L82 L83 L84 L85 L86 L87 | S163 S164 L88 L89 L90 S165 S166 S167 S168 L91 L92 L93 S169 S170 | L94 L95 L96 L97 L98 L99 L100 L101 L102 L103 L104 L105 L106
sketch "Sketch2" plane through (0, 254, 0) normal (0, 1, 0) x (1, 0, 0)
  line L0 (508, 508) -> (508, 19304) projected
  line L1 (35306, 19304) -> (35306, 508) projected
  line L2 (508, 19304) -> (35306, 19304)
  line L3 (35306, 19304) -> (35306, 508)
  line L4 (35306, 508) -> (508, 508)
  line L5 (508, 508) -> (508, 19304)
  point P0 (0, 0)
  constraints: 8 end point, 2 parallel, 1 horizontal, 1 perpendicular
sketch "Sketch3" plane through (0, 0, 0) normal (0, -1, 0) x (1, 0, 0)
  line L0 (508, -508) -> (508, -19304) projected
  line L1 (35306, -19304) -> (35306, -508) projected
  line L2 (508, -508) -> (35306, -508)
  line L3 (35306, -508) -> (35306, -19304)
  line L4 (35306, -19304) -> (508, -19304)
  line L5 (508, -19304) -> (508, -508)
  point P0 (0, 0)
  point P1 (35306, -508)
  constraints: 8 end point, 2 parallel, 1 horizontal, 1 perpendicular
extrude "Extrusion7" add sketch "Sketch3" against normal blind 279.4
extrude "Extrusion10" add sketch "Sketch1" along normal blind 254 separate body contours L3 L2 L1 L0
sketch "Sketch6" plane through (0, 254, 0) normal (0, 1, 0) x (1, 0, 0)
  line L0 (35560, 20135.0422) -> (75259.0076, 20135.0422)
  line L1 (75259.0076, 20135.0422) -> (75259.0076, -1959.9141)
  line L2 (75259.0076, -1959.9141) -> (35560, -1959.9141)
  line L3 (35560, -1959.9141) -> (35560, 20135.0422)
  point P0 (0, 0)
  constraints: 8 end point, 2 parallel, 1 horizontal, 1 perpendicular
extrude "Extrusion11" cut sketch "Sketch6" along normal mid plane 762 bodies 1
sketch "Sketch7" plane through (0, 254, 0) normal (0, 1, 0) x (1, 0, 0)
  line L0 (78604.4318, -257.3356) -> (35560, -257.3356)
  line L1 (35560, -257.3356) -> (35560, 23349.5653)
  line L2 (35560, 23349.5653) -> (78604.4318, 23349.5653)
  line L3 (78604.4318, 23349.5653) -> (78604.4318, -257.3356)
  point P0 (0, 0)
  constraints: 8 end point, 2 parallel, 1 horizontal, 1 perpendicular
extrude "Extrusion12" cut sketch "Sketch7" along normal mid plane 762 bodies 2
body "Solid1"
body "Solid3"
